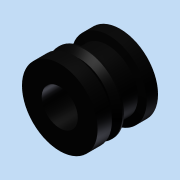
# Autodesk Inventor part: antenna_shaft_delrin
Saved by Autodesk Inventor 2014 (Build 180170000, 170)
## iProperties
Created: 2012-08-14
Part Number: antenna_shaft_delrin
Document SubType Name: Modeling
Designer: Robert Davis
Density: 1.425 g/cm^3
Material: Acetal Resin, Black
Mass: 0.0637251 g
Surface Area: 1.27177 cm^2
Volume: 0.0447194 cm^3
Appearance: Anodized - Black
Author: Robert Davis
Autodesk Inventor part; units mm, degrees
ref_plane "YZ Plane" through (0, 0, 0) normal (1, 0, 0) x (0, 1, 0)
ref_plane "XZ Plane" through (0, 0, 0) normal (0, 1, 0) x (-1, 0, 0)
ref_plane "XY Plane" through (0, 0, 0) normal (0, 0, 1) x (1, 0, 0)
sketch "Sketch1" plane through (0, 0, 0) normal (0, 0, 1) x (1, 0, 0)
  line L0 (0, 0) -> (0, 17.163)
  line L1 (2.5, 4) -> (2.5, 3.25)
  line L2 (2.5, 0) -> (0, 0)
  line L3 (2.5, 3.25) -> (2, 3.1618)
  line L4 (2, 3.1618) -> (2, 1.8382)
  line L5 (2, 1.8382) -> (2.5, 1.75)
  line L6 (0, 0) -> (0, 4)
  line L7 (0, 4) -> (2.5, 4)
  line L8 (2.5, 1.65) -> (2.15, 1.3)
  line L9 (2.15, 1.3) -> (2.5, 0.95)
  line L10 (2.5, 1.75) -> (2.5, 1.65)
  line L11 (2.5, 0.95) -> (2.5, 0)
  dimension "d2" = 5
  dimension "d17" = 0.75
  dimension "d18" = 1.75
  dimension "d19" = 100
  dimension "d20" = 100
  dimension "d24" = 1.3237
  dimension "d42" = 1.3
  dimension "d43" = 135
  dimension "d44" = 135
  dimension "d45" = 0.35
  constraints: 24 end point, 5 vertical, 2 collinear, 2 horizontal, 1 coincident
  measures "d2" diameter of L1 L0
  measures "d17" distance of L1.start L1.end
  measures "d18" distance of L5.end L2.start
  measures "d19" angle of L3 L4
  measures "d20" angle of L4 L5
  measures "d24" distance of L3.end L4.end
  measures "d42" distance from line of L2 L8.end
  measures "d43" angle of L10 L8
  measures "d44" angle of L11 L9
  measures "d45" distance from line of L11 L8.end
revolve "Revolution1" add sketch "Sketch1" angle 360 about axis through (0, 0, 0) along (0, 1, 0)
hole "Hole1" [suppressed]
hole "Hole2" at (0, 4, 0) direction (0, -1, 0) diameter 2.3876 end through all countersink diameter 4.7625 countersink angle 100
body "Solid1"
